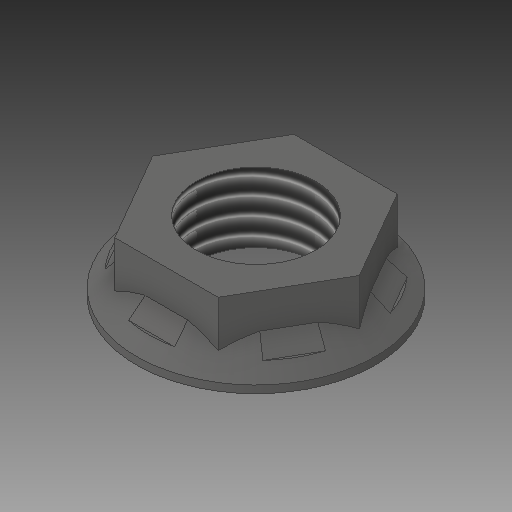
# Autodesk Inventor part: Nylon Nut
Saved by Autodesk Inventor 2019 (Build 230136000, 136)
## iProperties
Created: 2018-10-01
Part Number: Nylon Nut
Material: Generic
Document SubType Name: Modeling
Designer: Ax
Density: 1 g/cm^3
Appearance: Gray
Author: Ax
Autodesk Inventor part; units mm, degrees
ref_plane "YZ Plane" through (0, 0, 0) normal (1, 0, 0) x (0, 1, 0)
ref_plane "XZ Plane" through (0, 0, 0) normal (0, 1, 0) x (-1, 0, 0)
ref_plane "XY Plane" through (0, 0, 0) normal (0, 0, 1) x (1, 0, 0)
sketch "Sketch2" plane through (0, 0, 0) normal (0, 1, 0) x (-1, 0, 0)
  circle A0 centre (0, 0) radius 12
  dimension "d3" = 24
  constraints: 1 centre point
  measures "d3" diameter of A0
extrude "Extrusion1" add sketch "Sketch2" along normal blind 2
sketch "Sketch3" plane through (0, 2, 0) normal (0, 1, 0) x (1, 0, 0)
  line L0 (5.1962, 9) -> (10.3923, 0)
  line L1 (10.3923, 0) -> (5.1962, -9)
  line L2 (5.1962, -9) -> (-5.1962, -9)
  line L3 (-5.1962, -9) -> (-10.3923, 0)
  line L4 (-10.3923, 0) -> (-5.1962, 9)
  line L5 (-5.1962, 9) -> (5.1962, 9)
  point P0 (0, 0)
  point P1 (0, 0)
  dimension "d2" = 18
  constraints: 12 end point, 1 coincident, 1 horizontal, 13 other
  measures "d2" distance between parallel lines of L5 L2
extrude "Extrusion2" add sketch "Sketch3" along normal blind 5
chamfer "Chamfer1" distance 1.25 angle 45 1 edges at (12, 2, 0)
sketch "Sketch4" plane through (0, 7, 0) normal (0, 1, 0) x (1, 0, 0)
  circle A0 centre (0, 0) radius 6
  dimension "d9" = 12
  constraints: 1 centre point, 1 coincident
  measures "d9" diameter of A0
extrude "Extrusion3" cut sketch "Sketch4" against normal through all
chamfer "Chamfer2" distance 1.5 angle 45 6 edges at (7.7942, 2, 4.5) (7.7942, 2, -4.5) (0, 2, -9) (-7.7942, 2, -4.5) (0, 2, 9) (-7.7942, 2, 4.5)
thread "Thread1" size "M12x1.75" class "6H" standard "ISO Metric profile" full length
body "Solid1"
